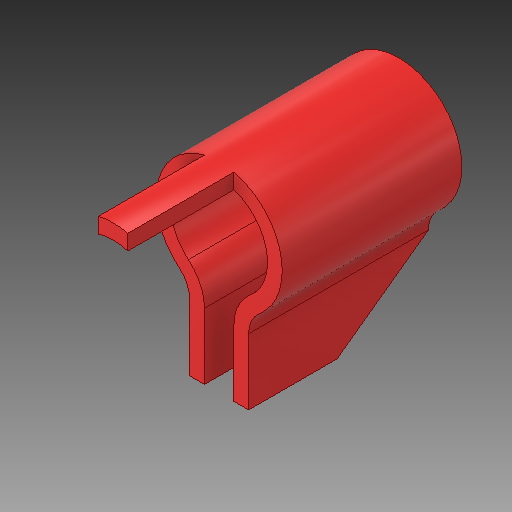
# Autodesk Inventor part: Part2
Saved by Autodesk Inventor 2019 (Build 230136000, 136)
## iProperties
Created: 2018-10-25
Part Number: Part2
Material: Iron, Gray
Document SubType Name: Sheet Metal
Designer: Isaac
Density: 7.15 g/cm^3
Flat Pattern Width: 4.85 cm
Flat Pattern Length: 7.87225 cm
Flat Pattern Area: 38.1804 cm^2
Sheet Metal Rule: Default_mm
Sheet Metal Width: 48.500 mm
Sheet Metal Length: 78.723 mm
Sheet Metal Area: 3818.043 mm^2
Appearance: Light Red
Author: Isaac
Autodesk Inventor part; units mm, degrees
ref_plane "YZ Plane" through (0, 0, 0) normal (1, 0, 0) x (0, 1, 0)
ref_plane "XZ Plane" through (0, 0, 0) normal (0, 1, 0) x (-1, 0, 0)
ref_plane "XY Plane" through (0, 0, 0) normal (0, 0, 1) x (1, 0, 0)
sketch "Sketch1" plane through (0, 0, 0) normal (0, 0, 1) x (1, 0, 0)
  line L0 (-5, -11.1967) -> (-5, 0)
  arc A0 (-5, 0) -> (-6.8153, 3.8546) centre (-10, 0) ccw
  arc A1 (6.8153, 3.8546) -> (-6.8153, 3.8546) centre (0, 12.1033) ccw
  arc A2 (6.8153, 3.8546) -> (5, 0) centre (10, 0) ccw
  line L1 (5, 0) -> (5, -11.1967)
  line L2 (-2.5, -11.1967) -> (-2.5, 0)
  arc A3 (-2.5, 0) -> (-5.2229, 5.7818) centre (-10, 0) ccw
  arc A4 (5.2229, 5.7818) -> (-5.2229, 5.7818) centre (0, 12.1033) ccw
  arc A5 (5.2229, 5.7818) -> (2.5, 0) centre (10, 0) ccw
  line L3 (2.5, 0) -> (2.5, -11.1967)
  line L4 (-5, -11.1967) -> (-2.5, -11.1967)
  line L5 (2.5, -11.1967) -> (5, -11.1967)
  point P0 (0, 0)
  dimension "d2" = 10.7
  dimension "d4" = 10
  dimension "d5" = 5
  dimension "d7" = 2.5
  dimension "d16" = 34
  constraints: 12 end point, 12 point on circle, 6 centre point, 4 horizontal alignment, 3 tangent, 2 vertical, 1 collinear, 1 equal radius, 1 horizontal, 1 vertical alignment, 4 other
  measures "d2" radius of A1
  measures "d4" distance of L1.end L0.start
  measures "d5" radius of A2
  measures "d7" radial gap between concentric circles of A1 A4
extrude "Extrusion1" add sketch "Sketch1" along normal blind 48.5
sketch "Sketch2" plane through (-5, -11.1967, 0) normal (0, -1, 0) x (1, 0, 0)
  line L0 (2.5, 0) -> (0, 0) projected
  line L1 (2.5, 0) -> (2.5, 48.5) projected
  line L2 (0, 48.5) -> (2.5, 48.5) projected
  line L3 (0, 0) -> (0, 48.5) projected
  line L4 (10, 0) -> (7.5, 0) projected
  line L5 (10, 0) -> (10, 48.5) projected
  line L6 (7.5, 48.5) -> (10, 48.5) projected
  line L7 (7.5, 0) -> (7.5, 48.5) projected
  line L8 (-5.7, 0) -> (-5.7, 48.5) projected
  line L9 (15.7, 0) -> (15.7, 48.5) projected
  line L10 (-5.7, 48.5) -> (2.5, 48.5)
  line L11 (2.5, 48.5) -> (2.5, 30.5)
  line L12 (2.5, 30.5) -> (-5.7, 30.5)
  line L13 (-5.7, 30.5) -> (-5.7, 48.5)
  line L14 (7.5, 48.5) -> (15.7, 48.5)
  line L15 (15.7, 48.5) -> (15.7, 30.5)
  line L16 (15.7, 30.5) -> (7.5, 30.5)
  line L17 (7.5, 30.5) -> (7.5, 48.5)
  point P0 (5, 0)
  point P1 (-1.6, 30.5)
  dimension "d10" = 18
  constraints: 16 end point, 4 parallel, 3 point on line, 2 horizontal, 2 perpendicular, 1 midpoint
  measures "d10" distance between parallel lines of L10 L12
extrude "Extrusion2" cut sketch "Sketch2" against normal blind 48.5 contours L12 L3 L2 L1 | L12 L8 L10 L3 | L16 L7 L6 L5 | L5 L14 L9 L16
sketch "Sketch3" plane through (5, -11.1967, 0) normal (1, 0, 0) x (0, 0, -1)
  line L0 (0, 0) -> (0, 11.1967)
  line L1 (0, 11.1967) -> (-15.5, 0)
  line L2 (-15.5, 0) -> (0, 0)
  line L3 (0, 11.1967) -> (0, 0) projected
  line L4 (0, 0) -> (-30.5, 0) projected
  dimension "d18" = 15.5
  constraints: 6 end point, 1 collinear, 1 perpendicular, 1 vertical
  measures "d18" distance of L1.end L0.start
extrude "Extrusion3" cut sketch "Sketch3" against normal blind 48.5
equation "\"BendRadius\" = Thickness"
equation "\"BendReliefWidth\" = Thickness"
equation "\"BendReliefDepth\" = 0.5 * Thickness"
equation "\"MinimumRemnant\" = 2 * Thickness"
equation "\"TransitionRadius\" = BendRadius"
equation "\"JacobiRadiusSize\" = BendRadius"
equation "\"GapSize\" = Thickness"
equation "\"Thickness\" = 2.5"
body "Solid1"
